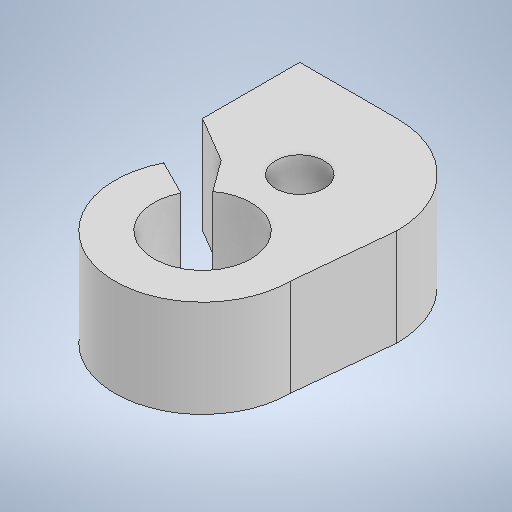
# Autodesk Inventor part: rod_exp1.1
Saved by Autodesk Inventor 2025 (Build 290162000, 162)
## iProperties
Created: 2024-06-29
Part Number: rod_exp1.1
Material: 一般
Document SubType Name: Modeling
Designer: Saigusa
Density: 1 g/cm^3
Appearance: 既定
Author: Saigusa
Autodesk Inventor part; units mm, degrees
ref_plane "YZ Plane" through (0, 0, 0) normal (1, 0, 0) x (0, 1, 0)
ref_plane "XZ Plane" through (0, 0, 0) normal (0, 1, 0) x (-1, 0, 0)
ref_plane "XY Plane" through (0, 0, 0) normal (0, 0, 1) x (1, 0, 0)
sketch "スケッチ1" plane through (0, 0, 0) normal (0, 1, 0) x (-1, 0, 0)
  line L0 (0, 0) -> (-5, 0)
  line L1 (-5, 0) -> (-5, 5)
  line L2 (-5, 5) -> (0, 5)
  line L3 (0, 5) -> (0, 0)
  circle A0 centre (-5, 5) radius 1.25
  line L4 (0, 0) -> (0, 15)
  circle A1 centre (-5, 5) radius 5
  circle A2 centre (-5, 5) radius 3
  line L5 (-8, 5) -> (-8, 0)
  line L6 (-8, 0) -> (-8, 15)
  line L7 (-8, 15) -> (0, 15)
  line L8 (-5, 5) -> (-5, 15)
  line L9 (-5, 10) -> (-8, 10)
  circle A3 centre (-5, 5) radius 2.25
  circle A4 centre (-5, 10) radius 2.5
  circle A5 centre (-5, 10) radius 4.5
  line L10 (-5, 10) -> (-0.9814, 7.975)
  line L11 (-5, 10) -> (-2.3337, 6.375)
  line L12 (-9.5, 10) -> (-10, 5)
  line L13 (-2.3337, 6.375) -> (-5, 10)
  line L14 (-5, 10) -> (-0.2269, 3.5108)
  line L15 (-0.2269, 3.5108) -> (-5, 0)
  line L16 (-2.3337, 6.375) -> (0, 5)
  point P0 (-3.5187, 7.9861)
  point P1 (-2.7674, 8.875)
  dimension "d0" = 5
  dimension "d1" = 5
  dimension "d2" = 2.5
  dimension "d3" = 15
  dimension "d4" = 6
  dimension "d5" = 4.5
  dimension "d8" = 5
  dimension "d10" = 9
  constraints: 34 end point, 10 point on circle, 6 centre point, 5 coincident, 5 point on line, 4 perpendicular, 3 equal length, 2 tangent, 2 vertical, 1 horizontal, 1 midpoint
  measures "d0" distance of L1.end L2.end
  measures "d1" distance of L0.end L1.end
  measures "d2" diameter of A0
  measures "d3" distance of L0.start L4.end
  measures "d4" diameter of A2
  measures "d5" diameter of A3
  measures "d8" diameter of A4
  measures "d10" diameter of A5
extrude "押し出し1" add sketch "スケッチ1" along normal blind 5 contours L0 A1 L3 | A1 L5 A2 L1 | L15 A1 | L1 A2 L2 L14 L15 | A1 L14 L2 | L2 L14 L16 | A2 A5 A3 L1 | L1 A3 L2 A2 | A1 L12 A5 L6 L5 | L2 A2 L14 | L10 A4 A1 | A1 A4 L8 A5 | A2 L2 A3 A5 | A5 A3 L8 A4 A2 L11 | A3 A5 A0 L1 | L1 A0 L2 A3 | L6 A5 A2 | A2 A4 L11 | A5 A0 L8 A3 | A3 L2 A0 A5 | A5 A2 A4 L8 A3 | A3 L8 A0 A5 | A5 L6 A1 A4 A2 | A5 A1 L6 | L12 A5 A1 | L8 A4 L9 L6 A5 | L6 L9 A4 A1 | A1 A5 L6 picked at (-1.7314, 8.4555)
sketch "スケッチ3" plane through (5, 0, 0) normal (0, 0, -1) x (-1, 0, 0)
  line L0 (5, 0) -> (5, 5) projected
  line L1 (5, 0) -> (2.5, 0)
  line L2 (2.5, 0) -> (2.5, 2.5)
  line L3 (2.5, 2.5) -> (5, 2.5)
  line L4 (5, 2.5) -> (5, 0)
  circle A0 centre (2.5, 2.5) radius 1.55
  dimension "d13" = 2.5
  dimension "d14" = 2.5
  dimension "d15" = 3.1
  constraints: 8 end point, 2 parallel, 1 centre point, 1 coincident, 1 horizontal, 1 perpendicular
  measures "d13" distance of L2.end L3.end
  measures "d14" distance of L1.end L2.end
  measures "d15" diameter of A0
extrude "押し出し2" cut sketch "スケッチ3" against normal blind 5 contours A0 L2 L3 | L3 L2 A0
